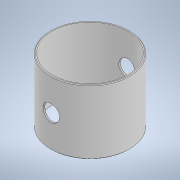
# Autodesk Inventor part: 75. Втулка шестерни третьей передачи
Saved by Autodesk Inventor 2021 (Build 250183000, 183)
## iProperties
Created: 2021-03-15
Part Number: 75. Втулка шестерни третьей передачи
Material: Типовые
Document SubType Name: Modeling
Designer: Данил
Density: 1 g/cm^3
Appearance: По умолчанию
Author: Данил
Autodesk Inventor part; units mm, degrees
ref_plane "YZ Plane" through (0, 0, 0) normal (1, 0, 0) x (0, 1, 0)
ref_plane "XZ Plane" through (0, 0, 0) normal (0, 1, 0) x (-1, 0, 0)
ref_plane "XY Plane" through (0, 0, 0) normal (0, 0, 1) x (1, 0, 0)
sketch "Эскиз1" plane through (0, 0, 0) normal (0, 0, 1) x (1, 0, 0)
  line L0 (0, 19.5) -> (0, -19.5)
  line L1 (23, -19.5) -> (23, 19.5)
  line L2 (23, 19.5) -> (23.6, 19.5)
  line L3 (24, 19.1) -> (24, -19.1)
  line L4 (23.6, -19.5) -> (23, -19.5)
  line L5 (24, -19.1) -> (23.6, -19.5)
  line L6 (24, 19.1) -> (23.6, 19.5)
  point P0 (0, 0)
  point P1 (0, 0)
  point P2 (24, 19.5)
  point P3 (24, -19.5)
  dimension "d0" = 39
  dimension "d1" = 48
  dimension "d2" = 46
  dimension "d7" = 0.4
  dimension "d8" = 45
  dimension "d9" = 0.4
  dimension "d10" = 45
  constraints: 14 end point, 4 point on line, 3 perpendicular, 2 horizontal alignment, 2 vertical, 1 coincident, 1 midpoint
  measures "d0" distance of L0.start L0.end
  measures "d1" diameter of L3 L0
  measures "d2" diameter of L1 L0
  measures "d7" distance of L3.end point (24, -19.5)
  measures "d8" angle of L3 L5
  measures "d9" distance of L3.start point (24, 19.5)
  measures "d10" angle of L3 L6
revolve "Вращение1" add sketch "Эскиз1" angle 360 about axis through (0, 19.5, 0) along (0, -1, 0)
sketch "Эскиз2" plane through (0, 0, 0) normal (0, 0, 1) x (1, 0, 0)
  circle A0 centre (0, 0) radius 5
  dimension "d4" = 10
  constraints: 1 centre point, 1 coincident
  measures "d4" diameter of A0
extrude "Выдавливание1" cut sketch "Эскиз2" along normal through all both and the other way through all
equation "\"d9\" = d7"
equation "\"d10\" = d8"
